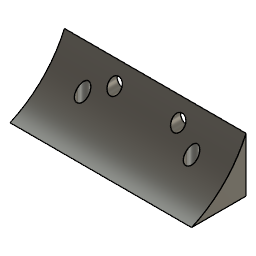
Soporte motor (Autodesk Fusion 360 design; units mm, degrees)
Autodesk Fusion 360 part; units mm, degrees
sketch "Boceto1" plane through (0, 0, 0) normal (1, 0, 0) x (0, 1, 0)
  line L0 (0, 0) -> (0, 15)
  line L1 (0, 0) -> (-15, 0)
  arc A0 (-15, 0) -> (0, 15) centre (-26.7073, 26.7073) ccw
  dimension "d1" = 15
  dimension "d2" = 15
  constraint coincident L0.start L1.start
  constraint vertical L0
  constraint perpendicular L0 L1
  measures "d1" distance of L0.start L0.end
  measures "d2" distance of L0.start L1.end
extrude "Extruir1" add sketch "Boceto1" along normal blind 50
sketch "Boceto2" plane through (0, 0, 0) normal (0, 1, 0) x (-1, 0, 0)
  line L0 (0, 0) -> (0, 15)
  line L1 (0, 15) -> (-50, 15)
  line L2 (-50, 15) -> (-50, 0)
  line L3 (-50, 0) -> (0, 0)
  circle A0 centre (-33.75, 10.6) radius 1.75
  circle A1 centre (-16.25, 10.6) radius 1.75
  dimension "d9" = 3.5
  dimension "d14" = 3.5
  measures "d9" diameter of A0
  measures "d14" diameter of A1
extrude "Extruir2" cut sketch "Boceto2" against normal blind 5 contours A0 | A1
sketch "Boceto3" plane through (0, 0, 0) normal (0, 0, -1) x (1, 0, 0)
  line L0 (0, 15) -> (0, 0)
  line L1 (0, 0) -> (50, 0)
  line L2 (50, 0) -> (50, 15)
  line L3 (50, 15) -> (0, 15)
  circle A0 centre (10, 5) radius 1.6
  circle A1 centre (40, 5) radius 1.6
  dimension "d19" = 3.2
  dimension "d22" = 3.2
  measures "d19" diameter of A0
  measures "d22" diameter of A1
extrude "Extruir3" cut sketch "Boceto3" against normal blind 11 contours A0 | A1
